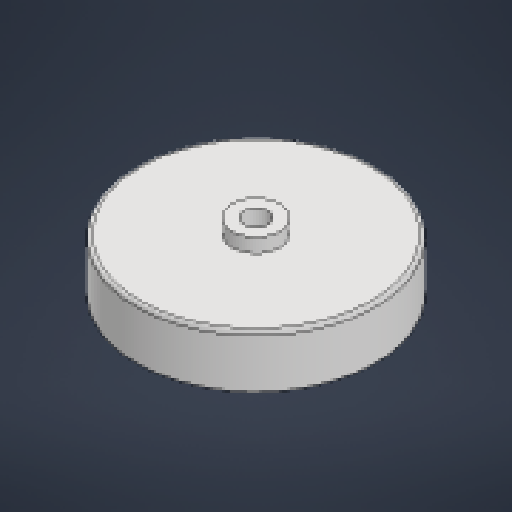
# Autodesk Inventor part: BIG-MAGNET
Saved by Autodesk Inventor 2026.1 (Build 301233020, 233B)
## iProperties
Created: 2026-03-20
Part Number: BIG-MAGNET
Material: Steel, Alloy
Document SubType Name: Modeling
Designer: Owen L
Mass: 174.805 g
Surface Area: 59.9348 cm^2
Volume: 22.6138 cm^3
Density: 7.73 g/cm^3
Appearance: Semi-Polished
Author: Owen L
Autodesk Inventor part; units mm, degrees
ref_plane "YZ Plane" through (0, 0, 0) normal (1, 0, 0) x (0, 1, 0)
ref_plane "XZ Plane" through (0, 0, 0) normal (0, 1, 0) x (-1, 0, 0)
ref_plane "XY Plane" through (0, 0, 0) normal (0, 0, 1) x (1, 0, 0)
sketch "Sketch1" plane through (0, 0, 0) normal (1, 0, 0) x (0, 1, 0)
  line L0 (0, 0) -> (0, 25.4)
  line L1 (0, 25.4) -> (11.1252, 25.4)
  line L2 (11.1252, 25.4) -> (11.1252, 5.1054)
  line L3 (11.1252, 5.1054) -> (14.097, 5.1054)
  line L4 (14.097, 5.1054) -> (14.097, 2.54)
  line L5 (14.097, 2.54) -> (6.35, 2.54)
  line L6 (6.35, 2.54) -> (6.35, 0)
  line L7 (6.35, 0) -> (0, 0)
  dimension "d1" = 11.1252
  dimension "d2" = 50.8
  dimension "d3" = 14.097
  dimension "d4" = 5.08
  dimension "d5" = 10.2108
  dimension "d6" = 6.35
  constraints: 16 end point, 7 perpendicular, 1 vertical
  measures "d1" distance of L0.end L1.end
  measures "d2" diameter of L1 L7
  measures "d3" distance between parallel lines of L0 L4
  measures "d4" diameter of L5 L7
  measures "d5" diameter of L3 L7
  measures "d6" distance between parallel lines of L0 L6
revolve "Revolution1" add sketch "Sketch1" angle 360 about axis through (0, 6.35, 0) along (0, -1, 0)
fillet "Fillet1" radius 0.7937 1 edges at (0, 11.1252, -25.4)
body "Solid1"
